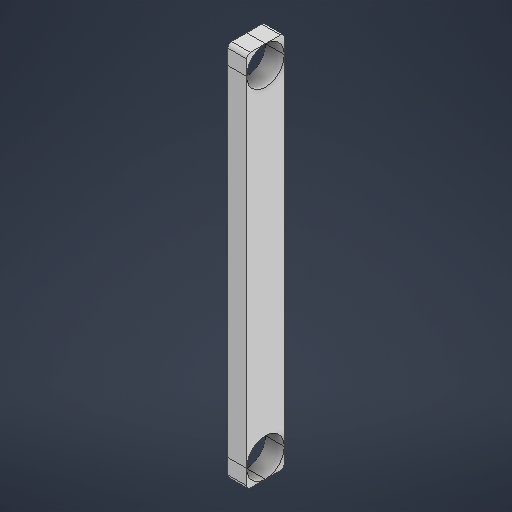
# Autodesk Inventor part: foot
Saved by Autodesk Inventor 2027 (Build 310192060, 192F)
## iProperties
Created: 2026-08-01
Part Number: foot
Material: Ogólny
Document SubType Name: Modeling
Designer: User
Density: 1 g/cm^3
Appearance: Domyślna
Author: User
Autodesk Inventor part; units mm, degrees
ref_plane "YZ Plane" through (0, 0, 0) normal (1, 0, 0) x (0, 1, 0)
ref_plane "XZ Plane" through (0, 0, 0) normal (0, 1, 0) x (-1, 0, 0)
ref_plane "XY Plane" through (0, 0, 0) normal (0, 0, 1) x (1, 0, 0)
sketch "Szkic1" plane through (0, 0, 0) normal (0, 1, 0) x (-1, 0, 0)
  line L0 (0.5, 1) -> (-0.5, 1)
  line L1 (-0.5, 1) -> (-0.5, -1)
  line L2 (-0.5, -1) -> (0.5, -1)
  line L3 (0.5, -1) -> (0.5, 1)
  line L4 (0.5, 1) -> (-0.5, -1) construction
  line L5 (-0.5, 1) -> (0.5, -1) construction
  point P0 (0, 0)
  dimension "d0" = 1
  dimension "d1" = 2
  constraints: 12 end point, 2 midpoint, 2 parallel, 1 horizontal, 1 perpendicular
  measures "d0" distance of L2.end L1.end
  measures "d1" distance of L1.end L0.end
extrude "Wyciągnięcie proste1" add sketch "Szkic1" along normal blind 20
sketch "Szkic2" plane through (0.5, 0, 1) normal (1, 0, 0) x (0, 0, -1)
  line L0 (0, 20) -> (2, 20) projected
  line L1 (1, 20) -> (1, 19)
  circle A0 centre (1, 19) radius 1
  line L2 (1, 0) -> (1, 1)
  circle A1 centre (1, 1) radius 1
  dimension "d5" = 1
  dimension "d6" = 2
  dimension "d10" = 1
  dimension "d11" = 2
  constraints: 4 end point, 2 centre point, 2 coincident, 2 vertical, 1 midpoint
  measures "d5" distance of L1.start L1.end
  measures "d6" diameter of A0
  measures "d10" distance of L2.start L2.end
  measures "d11" diameter of A1
extrude "Wyciągnięcie proste2" cut sketch "Szkic2" against normal blind 15
fillet "Zaokrąglenie2" radius 0.2 4 edges at (0, 0, 1) (0, 0, -1) (0, 20, 1) (0, 20, -1)
